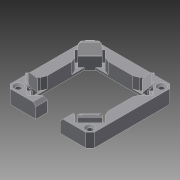
# Autodesk Inventor part: Держатель
Saved by Autodesk Inventor 2021.3 (Build 253353000, 353)
## iProperties
RuleStatus: InUse
Part Number: Держатель
Checked By: Якушев
Engr Approved By: Малов
Material: По умолчанию1
Document SubType Name: Modeling
Mfg Approved By: Судаков
Designer: Смирнов
Density: 1 g/cm^3
Appearance: По умолчанию1
AfterMaterialChange0: Материал
BeforeDocSave0: Материал
AfterAnyiPropertyChange0: Материал
Материал: По умолчанию1
Author: Смирнов
Autodesk Inventor part; units mm, degrees
ref_plane "YZ Plane" through (0, 0, 0) normal (1, 0, 0) x (0, 1, 0)
ref_plane "РабПлоскость1" through (0, 0, 0) normal (0, 0, -1) x (-1, 0, 0)
sketch "Эскиз1" plane through (0, 0, 0) normal (0, 0, -1) x (-1, 0, 0)
  line L0 (-21.1, -13.2716) -> (-21.1, 13.2716) construction
  line L1 (-21.1, -16.6858) -> (-21.1, 16.6858) construction
  arc A0 (-20.8071, 17.3929) -> (-21.1, 16.6858) centre (-20.1, 16.6858) ccw construction
  line L2 (-20.8071, 17.3929) -> (-17.3929, 20.8071) construction
  arc A1 (-16.6858, 21.1) -> (-17.3929, 20.8071) centre (-16.6858, 20.1) ccw construction
  line L3 (-16.6858, 21.1) -> (16.6858, 21.1) construction
  arc A2 (17.3929, 20.8071) -> (16.6858, 21.1) centre (16.6858, 20.1) ccw construction
  line L4 (17.3929, 20.8071) -> (20.8071, 17.3929) construction
  arc A3 (21.1, 16.6858) -> (20.8071, 17.3929) centre (20.1, 16.6858) ccw construction
  line L5 (17.3929, 20.8071) -> (20.8071, 17.3929) construction
  arc A4 (17.3929, 20.8071) -> (16.6858, 21.1) centre (16.6858, 20.1) ccw construction
  line L6 (-16.6858, 21.1) -> (16.6858, 21.1) construction
  arc A5 (-16.6858, 21.1) -> (-17.3929, 20.8071) centre (-16.6858, 20.1) ccw construction
  line L7 (-20.8071, 17.3929) -> (-17.3929, 20.8071) construction
  arc A6 (-20.8071, 17.3929) -> (-21.1, 16.6858) centre (-20.1, 16.6858) ccw construction
  line L8 (-21.1, -16.6858) -> (-21.1, 16.6858) construction
  arc A7 (-21.1, -16.6858) -> (-20.8071, -17.3929) centre (-20.1, -16.6858) ccw construction
  line L9 (-17.3929, -20.8071) -> (-20.8071, -17.3929) construction
  arc A8 (-17.3929, -20.8071) -> (-16.6858, -21.1) centre (-16.6858, -20.1) ccw construction
  line L10 (16.6858, -21.1) -> (-16.6858, -21.1) construction
  arc A9 (16.6858, -21.1) -> (17.3929, -20.8071) centre (16.6858, -20.1) ccw construction
  line L11 (20.8071, -17.3929) -> (17.3929, -20.8071) construction
  arc A10 (20.8071, -17.3929) -> (21.1, -16.6858) centre (20.1, -16.6858) ccw construction
  line L12 (21.1, 16.6858) -> (21.1, -16.6858) construction
  circle A11 centre (-15.35, -15.35) radius 0.2659 construction
  circle A12 centre (15.35, 15.35) radius 0.2659 construction
  circle A13 centre (-15.35, 15.35) radius 0.2659 construction
  circle A14 centre (15.35, -15.35) radius 0.2659 construction
  circle A15 centre (0, 0) radius 4 construction
  line L13 (17.3, -21.3) -> (-17.3, -21.3)
  line L14 (-21.3, -17.3) -> (-21.3, 17.3)
  line L15 (-17.3, 21.3) -> (17.3, 21.3)
  line L16 (21.3, 17.3) -> (21.3, -17.3)
  line L17 (21.3, -21.3) -> (-21.3, 21.3) construction
  line L18 (-21.3, -21.3) -> (21.3, 21.3) construction
  line L19 (-17.3, 21.3) -> (-21.3, 17.3)
  line L20 (21.3, 17.3) -> (17.3, 21.3)
  line L21 (21.3, -17.3) -> (17.3, -21.3)
  line L22 (-21.3, -17.3) -> (-17.3, -21.3)
  line L23 (-29.3, 29.3) -> (29.3, 29.3)
  line L24 (29.3, 29.3) -> (29.3, -29.3)
  line L25 (29.3, -29.3) -> (-29.3, -29.3)
  line L26 (-29.3, -29.3) -> (-29.3, 29.3)
  line L27 (-29.3, 29.3) -> (29.3, -29.3) construction
  line L28 (29.3, 29.3) -> (-29.3, -29.3) construction
  dimension "d0" = 0.2
  dimension "d1" = 4
  dimension "d2" = 4
  dimension "d3" = 4
  dimension "d4" = 4
  dimension "d5" = 4
  dimension "d6" = 4
  dimension "d7" = 4
  dimension "d8" = 4
  dimension "d12" = 8
  constraints: 32 end point, 9 point on line, 4 midpoint, 4 parallel, 3 perpendicular, 2 horizontal
  measures "d0" distance between parallel lines of L15 L6
  measures "d1" distance of L15.start L17.end
  measures "d2" distance of L14.end L17.end
  measures "d3" distance of L16.start L18.end
  measures "d4" distance of L15.end L18.end
  measures "d5" distance of L16.end L17.start
  measures "d6" distance of L13.start L17.start
  measures "d7" distance of L14.start L18.start
  measures "d8" distance of L13.end L18.start
  measures "d12" distance between parallel lines of L25 L13
extrude "Выдавливание1" add sketch "Эскиз1" against normal blind 10
ref_plane "РабПлоскость2" through (-19.3, -19.3, 10) normal (0.7071068, -0.7071068, 0) x (0, 0, -1)
sketch "Эскиз3" plane through (0, 0, 10) normal (0, 0, 1) x (1, 0, 0)
  line L0 (-17.3, -21.3) -> (-21.3, -17.3) construction
  line L1 (-21.3, -17.3) -> (-17.3, -21.3) construction
  line L2 (-17.3, -21.3) -> (-19.4213, -23.4213) construction
  line L3 (-19.4213, -23.4213) -> (-23.4213, -19.4213) construction
  line L4 (-23.4213, -19.4213) -> (-21.3, -17.3) construction
  line L5 (-21.3, -17.3) -> (-19.4213, -23.4213) construction
  line L6 (-17.3, -21.3) -> (-23.4213, -19.4213) construction
  line L7 (-23.0678, -12.4612) -> (-12.4612, -23.0678)
  line L8 (-12.4612, -23.0678) -> (-16.7038, -27.3104)
  line L9 (-16.7038, -27.3104) -> (-27.3104, -16.7038)
  line L10 (-27.3104, -16.7038) -> (-23.0678, -12.4612)
  line L11 (-23.0678, -12.4612) -> (-16.7038, -27.3104) construction
  line L12 (-12.4612, -23.0678) -> (-27.3104, -16.7038) construction
  line L13 (-29.3, -29.3) -> (-20.3607, -20.3607) construction
  line L14 (17.3, -21.3) -> (-17.3, -21.3) construction
  line L15 (-23.0678, -12.4612) -> (-19.8858, -9.2792)
  line L16 (-19.8858, -9.2792) -> (-9.2792, -19.8858)
  line L17 (-9.2792, -19.8858) -> (-12.4612, -23.0678)
  point P0 (0, 0)
  point P1 (-19.8858, -19.8858)
  point P2 (-19.8858, -19.8858)
  dimension "d13" = 3
  dimension "d14" = 5.6569
  dimension "d16" = 6
  dimension "d56" = 0.8284
  dimension "d57" = 15
  dimension "d58" = 4.5
  constraints: 32 end point, 6 perpendicular, 5 equal length, 5 midpoint, 2 collinear, 1 point on line
  measures "d13" distance of L3.end L0.end
  measures "d14" distance of L0.start L0.end
  measures "d16" distance of L7.end L8.end
  measures "d56" distance from line of L0 point (-19.886, -19.886)
  measures "d57" distance of L8.end L9.end
  measures "d58" distance between parallel lines of L7 L16
extrude "Выдавливание2" cut sketch "Эскиз3" against normal blind 8
chamfer "Фаска3" distance 2 angle 45 2 edges at (-21.3, -10.6934, 6) (-10.6934, -21.3, 6)
sketch "Эскиз4" plane through (-19.3, -19.3, 10) normal (0.7071068, -0.7071068, 0) x (0, 0, -1)
  line L0 (0.4, 0.3536) -> (0.4, 0.6464) construction
  line L1 (0.4, 24.173) -> (0.4, 0.6464) construction
  line L2 (9.5, 0.3536) -> (0.4, 0.3536) construction
  line L3 (10, 0) -> (8, 0) construction
  line L4 (8, 0) -> (0.5, 0)
  line L5 (0.5, 0) -> (0.0414, 1.5)
  line L6 (0.0414, 1.5) -> (-0.2586, 1.5)
  line L7 (-0.2586, 1.5) -> (-0.9285, -1)
  line L8 (-0.9285, -1) -> (8, -2)
  line L9 (8, 2.1716) -> (8, -3.8284) construction
  line L10 (8, -2) -> (8, 0)
  line L11 (-0.9285, -1) -> (-5, -5.0715)
  line L12 (-5, -5.0715) -> (-5, -3.2414)
  line L13 (-5, -3.2414) -> (-0.2586, 1.5)
  line L14 (0, -14.1421) -> (0, 27.2943) projected
  point P0 (10, 27.2943)
  dimension "d20" = 7.5
  dimension "d21" = 73
  dimension "d22" = 1.5
  dimension "d23" = 0.3
  dimension "d24" = 75
  dimension "d28" = 135
  dimension "d29" = 5
  dimension "d54" = 1.1464
  dimension "d55" = 1.2941
  dimension "d62" = 1
  dimension "d63" = 2
  constraints: 20 end point, 2 horizontal, 1 parallel, 1 perpendicular, 1 point on line, 1 vertical
  measures "d20" distance of L3.end L4.end
  measures "d21" angle of L4 L5
  measures "d22" distance between parallel lines of L4 L6
  measures "d23" distance of L5.end L6.end
  measures "d24" angle of L6 L7
  measures "d28" angle of L4 L11
  measures "d29" distance between parallel lines of L14 L12
  measures "d54" distance between parallel lines of L6 L2
  measures "d55" distance between parallel lines of L11 L13
  measures "d62" distance from line of L4 L7.end
  measures "d63" distance of L8.end L3.end
extrude "Выдавливание3" add sketch "Эскиз4" along normal mid plane 12
fillet "Сопряжение4" radius 2 2 edges at (-17.9964, -26.4817, 15) (-26.4817, -17.9964, 15)
fillet "Сопряжение2" radius 0.2 2 edges at (-20.7142, -20.7142, 2) (-22.0071, -22.0071, 2)
fillet "Сопряжение5" radius 0.3 5 edges at (-18.6435, -26.3003, 14.4142) (-16.4969, -24.9821, 11.9642) (-26.3003, -18.6435, 14.4142) (-24.9821, -16.4969, 11.9642) (-22.8861, -22.8861, 15)
pattern_circular "Круговой массив2" count 4 over 360 about axis through (0, 0, -10) along (0, 0, 1) of "Выдавливание2", "Выдавливание3", "Сопряжение4", "Сопряжение2", "Сопряжение5"
chamfer "Фаска4" distance 2 angle 45 6 edges at (-21.3, 10.6934, 6) (-10.6934, 21.3, 6) (10.6934, -21.3, 6) (21.3, -10.6934, 6) (21.3, 10.6934, 6) (10.6934, 21.3, 6)
sketch "Эскиз5" plane through (0, 0, 10) normal (0, 0, 1) x (1, 0, 0)
  line L0 (-25, -25) -> (25, -25) construction
  line L1 (25, -25) -> (25, 25) construction
  line L2 (25, 25) -> (-25, 25) construction
  line L3 (-25, 25) -> (-25, -25) construction
  line L4 (-25, -25) -> (25, 25) construction
  line L5 (25, -25) -> (-25, 25) construction
  point P0 (0, 0)
  dimension "d37" = 50
  constraints: 12 end point, 4 coincident, 2 midpoint, 2 parallel, 2 perpendicular, 1 horizontal
  measures "d37" distance of L0.start L0.end
hole "Отверстие1" at (25, 25, 10) at (25, -25, 10) at (-25, -25, 10) at (-25, 25, 10) direction (0, 0, -1) diameter 3.4 end through all countersink diameter 6 countersink angle 90 clearance for "с потайной головкой ГОСТ 12876-67" size "M3" standard "ГОСТ"
chamfer "Фаска1" distance 3 angle 45 4 edges at (29.3, -29.3, 5) (-29.3, -29.3, 5) (-29.3, 29.3, 5) (29.3, 29.3, 5)
sketch "Эскиз6" plane through (0, 0, 10) normal (0, 0, 1) x (1, 0, 0)
  line L0 (0, 0) -> (0, -43.6922) construction
  line L1 (-16.6858, -21.1) -> (16.6858, -21.1) construction
  line L2 (-26.3, -29.3) -> (26.3, -29.3) construction
  line L3 (-8.5, -21.1) -> (8.5, -21.1)
  line L4 (8.5, -21.1) -> (8.5, -29.3)
  line L5 (8.5, -29.3) -> (-8.5, -29.3)
  line L6 (-8.5, -29.3) -> (-8.5, -21.1)
  dimension "d48" = 17
  constraints: 10 end point, 2 parallel, 1 collinear, 1 horizontal, 1 perpendicular, 1 point on line, 1 vertical, 1 other
  measures "d48" distance between parallel lines of L4 L6
extrude "Выдавливание4" cut sketch "Эскиз6" against normal through all
chamfer "Фаска2" distance 2 angle 45 2 edges at (-8.5, -25.3, 10) (8.5, -25.3, 10)
sketch "Эскиз7" plane through (0, 0, 0) normal (0, 0, -1) x (-1, 0, 0)
  line L0 (-8.5, -29.3) -> (-8.5, -21.3) projected
  line L1 (-8.5, -21.3) -> (-17.3, -21.3) projected
  line L2 (-17.3, -21.3) -> (-21.3, -17.3) projected
  line L3 (-21.3, -17.3) -> (-21.3, 17.3) projected
  line L4 (-21.3, 17.3) -> (-17.3, 21.3) projected
  line L5 (-17.3, 21.3) -> (17.3, 21.3) projected
  line L6 (17.3, 21.3) -> (21.3, 17.3) projected
  line L7 (21.3, 17.3) -> (21.3, -17.3) projected
  line L8 (21.3, -17.3) -> (17.3, -21.3) projected
  line L9 (17.3, -21.3) -> (8.5, -21.3) projected
  line L10 (8.5, -21.3) -> (8.5, -29.3) projected
  line L11 (8.5, -29.3) -> (26.3, -29.3) projected
  line L12 (29.3, -26.3) -> (26.3, -29.3) projected
  line L13 (29.3, -26.3) -> (29.3, 26.3) projected
  line L14 (26.3, 29.3) -> (29.3, 26.3) projected
  line L15 (26.3, 29.3) -> (-26.3, 29.3) projected
  line L16 (-29.3, 26.3) -> (-26.3, 29.3) projected
  line L17 (-29.3, 26.3) -> (-29.3, -26.3) projected
  line L18 (-26.3, -29.3) -> (-29.3, -26.3) projected
  line L19 (-26.3, -29.3) -> (-8.5, -29.3) projected
  circle A0 centre (25, -25) radius 1.7 projected
  circle A1 centre (-25, 25) radius 1.7 projected
  circle A2 centre (-25, -25) radius 1.7 projected
  circle A3 centre (25, 25) radius 1.7 projected
  point P0 (0, 0)
extrude "Выдавливание5" cut sketch "Эскиз7" against normal blind 0.5
sketch "Эскиз8" plane through (0, 0, 0.5) normal (0, 0, -1) x (-1, 0, 0)
  circle A0 centre (25, -25) radius 1.7 construction
  circle A1 centre (-25, -25) radius 1.7 construction
  circle A2 centre (-25, 25) radius 1.7 construction
  circle A3 centre (25, 25) radius 1.7 construction
  point P0 (0, 0)
hole "Отверстие2" at (-25, -25, 0.5) at (-25, 25, 0.5) at (25, -25, 0.5) at (25, 25, 0.5) direction (0, 0, 1) diameter 3.9 depth 5 countersink diameter 4.5 countersink angle 90
equation "\"d2\" = d1"
equation "\"d4\" = d3"
equation "\"d5\" = d3"
equation "\"d6\" = d5"
equation "\"d7\" = d3"
equation "\"d8\" = d7"
